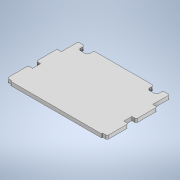
# Autodesk Inventor part: back_wall
Saved by Autodesk Inventor 2020 (Build 240168000, 168)
## iProperties
Created: 2019-06-12
Part Number: back_wall
Material: Generic
Document SubType Name: Modeling
Designer: Dammy
Density: 1 g/cm^3
Appearance: Default
Author: Dammy
Autodesk Inventor part; units mm, degrees
ref_plane "YZ Plane" through (0, 0, 0) normal (1, 0, 0) x (0, 1, 0)
ref_plane "XZ Plane" through (0, 0, 0) normal (0, 1, 0) x (-1, 0, 0)
ref_plane "XY Plane" through (0, 0, 0) normal (0, 0, 1) x (1, 0, 0)
sketch "Sketch1" plane through (0, 0, 0) normal (0, 1, 0) x (-1, 0, 0)
  line L0 (-2, -70.675) -> (-6, -70.675)
  line L1 (-6, -41.675) -> (-2, -41.675)
  line L2 (0, -43.675) -> (0, -68.675)
  line L3 (-6, -30.675) -> (-2, -30.675)
  line L4 (0, -28.675) -> (0, -3.675)
  line L5 (-2, -1.675) -> (-6, -1.675)
  arc A0 (0, -3.675) -> (-2, -1.675) centre (-2, -3.675) ccw
  arc A1 (-2, -30.675) -> (0, -28.675) centre (-2, -28.675) ccw
  arc A2 (0, -43.675) -> (-2, -41.675) centre (-2, -43.675) ccw
  arc A3 (-2, -70.675) -> (0, -68.675) centre (-2, -68.675) ccw
  line L6 (-136.5, -70.675) -> (-132.5, -70.675)
  line L7 (-132.5, -41.675) -> (-136.5, -41.675)
  line L8 (-138.5, -43.675) -> (-138.5, -68.675)
  line L9 (-136.5, -30.675) -> (-132.5, -30.675)
  line L10 (-132.5, -1.675) -> (-136.5, -1.675)
  line L11 (-138.5, -3.675) -> (-138.5, -28.675)
  arc A4 (-136.5, -1.675) -> (-138.5, -3.675) centre (-136.5, -3.675) ccw
  arc A5 (-138.5, -28.675) -> (-136.5, -30.675) centre (-136.5, -28.675) ccw
  arc A6 (-136.5, -41.675) -> (-138.5, -43.675) centre (-136.5, -43.675) ccw
  arc A7 (-138.5, -68.675) -> (-136.5, -70.675) centre (-136.5, -68.675) ccw
  line L12 (-27.75, -91) -> (-27.75, -88)
  line L13 (-110.75, -91) -> (-110.75, -88)
  line L14 (-30.75, -94) -> (-107.75, -94)
  line L15 (0, -56.175) -> (-138.5, -56.175) construction
  line L16 (-113.75, -85) -> (-120.45, -85)
  line L17 (-123.45, -88) -> (-123.45, -91)
  line L18 (-126.45, -94) -> (-127.7679, -94)
  line L19 (-24.75, -85) -> (-18.05, -85)
  line L20 (-15.05, -88) -> (-15.05, -91)
  line L21 (-12.05, -94) -> (-8, -94)
  arc A8 (-15.05, -91) -> (-12.05, -94) centre (-12.05, -91) ccw
  arc A9 (-15.05, -88) -> (-18.05, -85) centre (-18.05, -88) ccw
  arc A10 (-24.75, -85) -> (-27.75, -88) centre (-24.75, -88) ccw
  arc A11 (-30.75, -94) -> (-27.75, -91) centre (-30.75, -91) ccw
  arc A12 (-110.75, -91) -> (-107.75, -94) centre (-107.75, -91) ccw
  arc A13 (-110.75, -88) -> (-113.75, -85) centre (-113.75, -88) ccw
  arc A14 (-120.45, -85) -> (-123.45, -88) centre (-120.45, -88) ccw
  arc A15 (-126.45, -94) -> (-123.45, -91) centre (-126.45, -91) ccw
  line L22 (-7.5, 0) -> (-128.9984, 0)
  line L23 (-6, -70.675) -> (-6, -92)
  line L24 (-6, -30.675) -> (-6, -41.675)
  line L25 (-132.5, -30.675) -> (-132.5, -41.675)
  line L26 (-132.5, -70.675) -> (-132.5, -91)
  line L27 (-128.9984, 0) -> (-131.5, 0)
  line L28 (-132.5, -1) -> (-132.5, -1.675)
  arc A16 (-131.5, 0) -> (-132.5, -1) centre (-131.5, -1) ccw
  line L29 (-6, -1.675) -> (-6, -1)
  line L30 (-6, 0) -> (-6, 0)
  line L31 (-7, 0) -> (-7.5, 0)
  arc A17 (-6, -1) -> (-7, 0) centre (-7, -1) ccw
  line L32 (-132.5, -91) -> (-132.5, -92)
  line L33 (-130.5, -94) -> (-127.109, -94)
  arc A18 (-132.5, -92) -> (-130.5, -94) centre (-130.5, -92) ccw
  line L34 (-4.5, -94) -> (-10.025, -94)
  arc A19 (-8, -94) -> (-6, -92) centre (-8, -92) ccw
  point P0 (0, 0)
  point P1 (0, -70.675)
  point P2 (-4, -70.675)
  point P3 (-138.5, -41.675)
  point P4 (-138.5, -30.675)
  point P5 (-134.5, -70.675)
  point P6 (-132.5, -94)
  point P7 (-27.75, -94)
  point P8 (-27.75, -85)
  point P9 (-110.75, -94)
  point P10 (-110.75, -85)
  point P11 (-69.25, -94)
  point P12 (-69.25, -56.175)
  point P13 (-123.45, -85)
  point P14 (-15.05, -85)
  point P15 (-6.4873, -94)
  point P16 (-6, -91.775)
  point P17 (-4, -1.675)
  point P18 (-134.5, -1.675)
  point P19 (0, -16.175)
  point P20 (-6, -81.3375)
  point P21 (-6, -36.175)
  point P22 (-132.5, -80.8375)
  point P23 (-132.5, -36.175)
  point P24 (-138.5, -16.175)
  point P25 (-132.5, -1.3375)
  dimension "d3" = 6
  dimension "d8" = 2
  dimension "d11" = 2
  dimension "d12" = 2
  dimension "d13" = 9
  dimension "d14" = 83
  dimension "d15" = 12.7
  dimension "d16" = 12.7
  dimension "d18" = 3
  dimension "d19" = 3
  dimension "d23" = 94.0001
  dimension "d24" = 6
  dimension "d25" = 1
  dimension "d26" = 1
  dimension "d29" = 29
  dimension "d30" = 23.325
  dimension "d31" = 2
  dimension "d32" = 69
  dimension "d33" = 11
  dimension "d34" = 2
  dimension "d35" = 126.5
  constraints: 70 end point, 40 point on circle, 40 tangent, 28 point on line, 20 centre point, 17 midpoint, 13 vertical alignment, 11 equal radius, 9 horizontal, 9 horizontal alignment, 6 parallel, 6 perpendicular, 6 vertical, 3 collinear
  measures "d3" distance of point (0, -70.675) L0.end
  measures "d8" radius of A0
  measures "d11" radius of A4
  measures "d12" radius of A6
  measures "d13" distance of point (-27.75, -94) point (-27.75, -85)
  measures "d14" distance between parallel lines of L13 L12
  measures "d15" distance of point (-110.75, -85) point (-123.45, -85)
  measures "d16" distance of point (-27.75, -85) point (-15.05, -85)
  measures "d18" radius of A8
  measures "d19" radius of A12
  measures "d23" distance between parallel lines of L22 L14
  measures "d24" distance between parallel lines of L8 L26
  measures "d25" radius of A16
  measures "d26" radius of A17
  measures "d29" distance from line of L1 point (-4, -70.675)
  measures "d30" distance from line of L21 point (-4, -70.675)
  measures "d31" radius of A18
  measures "d32" distance between parallel lines of L5 L0
  measures "d33" distance between parallel lines of L3 L1
  measures "d34" radius of A19
  measures "d35" distance between parallel lines of L26 L23
extrude "Extrusion1" add sketch "Sketch1" along normal blind 5
equation "\"d19\" = d18"
equation "\"d24\" = d3"
equation "\"d25\" = d26"
equation "\"d31\" = d17"
equation "\"d33\" = d32 - 2 * d29"
equation "\"d17\" = 2"
body "Solid1"
